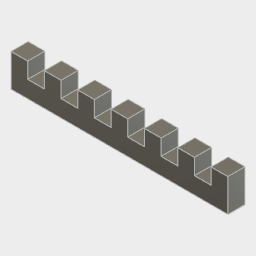
FingerActuator v4 (Autodesk Fusion 360 design; units mm, degrees)
Autodesk Fusion 360 part; units mm, degrees
sketch "Sketch1" plane through (0, 0, 0) normal (0, 1, 0) x (1, 0, 0)
  line L0 (0, 0) -> (88, 0)
  line L1 (88, 0) -> (88, 8.2)
  line L2 (88, 8.2) -> (0, 8.2)
  line L3 (0, 8.2) -> (0, 0)
  dimension "d1" = 88
  dimension "d2" = 8.2
  measures "d1" distance of L0.start L0.end
  measures "d2" distance of L0.start L2.end
sketch "Sketch2" plane through (0, 12.75, 0) normal (0, 1, 0) x (-1, 0, 0)
  line L0 (0, -8.2) -> (0, 0)
  line L1 (0, 0) -> (-88, 0)
  line L2 (-88, 0) -> (-88, -8.2)
  line L3 (-88, -8.2) -> (0, -8.2)
  line L4 (0, 0) -> (-6.77, 0)
  line L5 (-6.77, 0) -> (-6.77, -8.2)
  line L6 (-6.77, -8.2) -> (0, -8.2)
  line L7 (0, -8.2) -> (0, 0)
  line L8 (-6.77, -8.2) -> (-13.54, -8.2)
  line L9 (-13.54, -8.2) -> (-13.54, 0)
  line L10 (-13.54, 0) -> (-6.77, 0)
  line L11 (-6.77, 0) -> (-6.77, -8.2)
  dimension "d5" = 6.77
  dimension "d6" = 6.77
  measures "d5" distance of L0.end L4.end
  measures "d6" distance of L5.end L8.end
sketch "Sketch3" plane through (0, 12.75, 0) normal (0, 1, 0) x (-1, 0, 0)
  line L0 (-13.54, -8.2) -> (-13.54, 0)
  line L1 (-13.54, 0) -> (-88, 0)
  line L2 (-88, 0) -> (-88, -8.2)
  line L3 (-88, -8.2) -> (-13.54, -8.2)
  line L4 (-13.54, 0) -> (-20.31, 0)
  line L5 (-20.31, 0) -> (-20.31, -8.2)
  line L6 (-20.31, -8.2) -> (-13.54, -8.2)
  line L7 (-13.54, -8.2) -> (-13.54, 0)
  line L8 (-20.31, -8.2) -> (-27.08, -8.2)
  line L9 (-27.08, -8.2) -> (-27.08, 0)
  line L10 (-27.08, 0) -> (-20.31, 0)
  line L11 (-20.31, 0) -> (-20.31, -8.2)
  dimension "d9" = 6.77
  dimension "d10" = 6.77
  measures "d9" distance of L0.end L4.end
  measures "d10" distance of L5.end L8.end
sketch "Sketch4" plane through (0, 12.75, 0) normal (0, 1, 0) x (-1, 0, 0)
  line L0 (-27.08, -8.2) -> (-27.08, 0)
  line L1 (-27.08, 0) -> (-88, 0)
  line L2 (-88, 0) -> (-88, -8.2)
  line L3 (-88, -8.2) -> (-27.08, -8.2)
  line L4 (-27.08, 0) -> (-33.85, 0)
  line L5 (-33.85, 0) -> (-33.85, -8.2)
  line L6 (-33.85, -8.2) -> (-27.08, -8.2)
  line L7 (-27.08, -8.2) -> (-27.08, 0)
  line L8 (-33.85, -8.2) -> (-40.62, -8.2)
  line L9 (-40.62, -8.2) -> (-40.62, 0)
  line L10 (-40.62, 0) -> (-33.85, 0)
  line L11 (-33.85, 0) -> (-33.85, -8.2)
  dimension "d13" = 6.77
  dimension "d14" = 6.77
  measures "d13" distance of L0.end L4.end
  measures "d14" distance of L5.end L8.end
sketch "Sketch5" plane through (0, 12.75, 0) normal (0, 1, 0) x (-1, 0, 0)
  line L0 (-40.62, -8.2) -> (-40.62, 0)
  line L1 (-40.62, 0) -> (-88, 0)
  line L2 (-88, 0) -> (-88, -8.2)
  line L3 (-88, -8.2) -> (-40.62, -8.2)
  line L4 (-40.62, 0) -> (-47.39, 0)
  line L5 (-47.39, 0) -> (-47.39, -8.2)
  line L6 (-47.39, -8.2) -> (-40.62, -8.2)
  line L7 (-40.62, -8.2) -> (-40.62, 0)
  line L8 (-47.39, -8.2) -> (-54.16, -8.2)
  line L9 (-54.16, -8.2) -> (-54.16, 0)
  line L10 (-54.16, 0) -> (-47.39, 0)
  line L11 (-47.39, 0) -> (-47.39, -8.2)
  dimension "d17" = 6.77
  dimension "d18" = 6.77
  measures "d17" distance of L0.end L4.end
  measures "d18" distance of L5.end L8.end
sketch "Sketch6" plane through (0, 12.75, 0) normal (0, 1, 0) x (-1, 0, 0)
  line L0 (-54.16, -8.2) -> (-54.16, 0)
  line L1 (-54.16, 0) -> (-88, 0)
  line L2 (-88, 0) -> (-88, -8.2)
  line L3 (-88, -8.2) -> (-54.16, -8.2)
  line L4 (-54.16, 0) -> (-60.93, 0)
  line L5 (-60.93, 0) -> (-60.93, -8.2)
  line L6 (-60.93, -8.2) -> (-54.16, -8.2)
  line L7 (-54.16, -8.2) -> (-54.16, 0)
  line L8 (-60.93, 0) -> (-67.7, 0)
  line L9 (-67.7, 0) -> (-67.7, -8.2)
  line L10 (-67.7, -8.2) -> (-60.93, -8.2)
  line L11 (-60.93, -8.2) -> (-60.93, 0)
  dimension "d21" = 6.77
  dimension "d22" = 6.77
  measures "d21" distance of L0.end L4.end
  measures "d22" distance of L4.end L8.end
sketch "Sketch7" plane through (0, 12.75, 0) normal (0, 1, 0) x (-1, 0, 0)
  line L0 (-67.7, -8.2) -> (-67.7, 0)
  line L1 (-67.7, 0) -> (-88, 0)
  line L2 (-88, 0) -> (-88, -8.2)
  line L3 (-88, -8.2) -> (-67.7, -8.2)
  line L4 (-67.7, 0) -> (-74.47, 0)
  line L5 (-74.47, 0) -> (-74.47, -8.2)
  line L6 (-74.47, -8.2) -> (-67.7, -8.2)
  line L7 (-67.7, -8.2) -> (-67.7, 0)
  line L8 (-74.47, -8.2) -> (-81.24, -8.2)
  line L9 (-81.24, -8.2) -> (-81.24, 0)
  line L10 (-81.24, 0) -> (-74.47, 0)
  line L11 (-74.47, 0) -> (-74.47, -8.2)
  dimension "d25" = 6.77
  dimension "d26" = 6.77
  measures "d25" distance of L0.end L4.end
  measures "d26" distance of L5.end L8.end
sketch "Sketch8" plane through (0, 0, 0) normal (0, 1, 0) x (1, 0, 0)
sketch "Sketch9" plane through (0, 0, 0) normal (0, 1, 0) x (1, 0, 0)
  line L0 (0, -10) -> (88.9, -10)
  line L1 (88.9, -10) -> (88.9, -17.02)
  line L2 (88.9, -17.02) -> (0, -17.02)
  line L3 (0, -17.02) -> (0, -10)
  dimension "d32" = 88.9
  dimension "d33" = 7.02
  measures "d32" distance of L0.start L0.end
  measures "d33" distance of L0.start L2.end
extrude "Extrude9" add sketch "Sketch9" along normal blind 13.47
sketch "Sketch10" plane through (0, 13.47, 0) normal (0, 1, 0) x (-1, 0, 0)
  line L0 (0, 17.02) -> (-88.9, 17.02)
  line L1 (-88.9, 17.02) -> (-88.9, 10)
  line L2 (-88.9, 10) -> (0, 10)
  line L3 (0, 10) -> (0, 17.02)
  line L4 (-6.8385, 17.02) -> (-13.6769, 17.02)
  line L5 (-13.6769, 17.02) -> (-13.6769, 10)
  line L6 (-13.6769, 10) -> (-6.8385, 10)
  line L7 (-6.8385, 10) -> (-6.8385, 17.02)
  line L8 (-20.5154, 17.02) -> (-27.3538, 17.02)
  line L9 (-27.3538, 17.02) -> (-27.3538, 10)
  line L10 (-27.3538, 10) -> (-20.5154, 10)
  line L11 (-20.5154, 10) -> (-20.5154, 17.02)
  line L12 (-34.1923, 17.02) -> (-41.0308, 17.02)
  line L13 (-41.0308, 17.02) -> (-41.0308, 10)
  line L14 (-41.0308, 10) -> (-34.1923, 10)
  line L15 (-34.1923, 10) -> (-34.1923, 17.02)
  line L16 (-47.8692, 17.02) -> (-54.7077, 17.02)
  line L17 (-54.7077, 17.02) -> (-54.7077, 10)
  line L18 (-54.7077, 10) -> (-47.8692, 10)
  line L19 (-47.8692, 10) -> (-47.8692, 17.02)
  line L20 (-61.5462, 17.02) -> (-68.3846, 17.02)
  line L21 (-68.3846, 17.02) -> (-68.3846, 10)
  line L22 (-68.3846, 10) -> (-61.5462, 10)
  line L23 (-61.5462, 10) -> (-61.5462, 17.02)
  line L24 (-75.2231, 17.02) -> (-82.0615, 17.02)
  line L25 (-82.0615, 17.02) -> (-82.0615, 10)
  line L26 (-82.0615, 10) -> (-75.2231, 10)
  line L27 (-75.2231, 10) -> (-75.2231, 17.02)
  point P0 (0, 17.02)
  point P1 (-6.8385, 17.02)
  point P2 (-13.6769, 17.02)
  point P3 (-20.5154, 17.02)
  point P4 (-27.3538, 17.02)
  point P5 (-34.1923, 17.02)
  point P6 (-41.0308, 17.02)
  point P7 (-47.8692, 17.02)
  point P8 (-54.7077, 17.02)
  point P9 (-61.5462, 17.02)
  point P10 (-68.3846, 17.02)
  point P11 (-75.2231, 17.02)
  point P12 (-82.0615, 17.02)
  point P13 (-88.9, 17.02)
  dimension "d38" = 88.9
  dimension "d39" = 0
  dimension "d40" = 6.8385
  dimension "d43" = 6.8385
  dimension "d46" = 6.8385
  dimension "d47" = 6.8385
  dimension "d48" = 6.8385
  dimension "d49" = 7.02
  dimension "d50" = 6.8385
  measures "d40" distance of P1 P2
  measures "d43" distance of P3 P4
  measures "d46" distance of P5 P6
  measures "d47" distance of P7 P8
  measures "d48" distance of P9 P10
  measures "d49" distance of P9 L22.end
  measures "d50" distance of P11 P12
extrude "Extrude12" cut sketch "Sketch10" against normal blind 6.5 contours L0 L2 L4 L5 L6 L7
extrude "Extrude11" cut sketch "Sketch10" against normal blind 6.5 contours L0 L2 L4 L5 L6 L7
extrude "Extrude10" cut sketch "Sketch10" against normal blind 6.5 contours L0 L2 L4 L5 L6 L7
extrude "Extrude13" cut sketch "Sketch10" against normal blind 6.5 contours L0 L2 L8 L9 L10 L11
extrude "Extrude14" cut sketch "Sketch10" against normal blind 6.5 contours L0 L2 L12 L13 L14 L15
extrude "Extrude15" cut sketch "Sketch10" against normal blind 6.5 contours L0 L2 L16 L17 L18 L19
extrude "Extrude16" cut sketch "Sketch10" against normal blind 6.5 contours L0 L2 L20 L21 L22 L23
extrude "Extrude17" cut sketch "Sketch10" against normal blind 6.5 contours L0 L2 L24 L25 L26 L27
